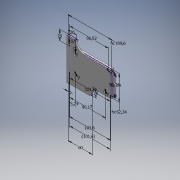
# Autodesk Inventor part: support arduino_v2
Saved by Autodesk Inventor 2016 (Build 200138000, 138)
## iProperties
Created: 2018-12-12
Part Number: support arduino_v2
Material: Generic
Document SubType Name: Modeling
Designer: Mick
Density: 1 g/cm^3
Appearance: Default
Author: Mick
Autodesk Inventor part; units mm, degrees
note: some values were not read from the file. Chosen so that the rebuilt part matches the saved one: edges of "Fillet3".
ref_plane "YZ Plane" through (0, 0, 0) normal (1, 0, 0) x (0, 1, 0)
ref_plane "XZ Plane" through (0, 0, 0) normal (0, 1, 0) x (-1, 0, 0)
ref_plane "XY Plane" through (0, 0, 0) normal (0, 0, 1) x (1, 0, 0)
sketch "Sketch1" plane through (0, 0, 0) normal (0, 1, 0) x (-1, 0, 0)
  line L0 (-50.8, 26.67) -> (-50.8, -26.67)
  line L1 (-50.8, -26.67) -> (50.8, -26.67)
  line L2 (50.8, -26.67) -> (50.8, 26.67)
  line L3 (50.8, 26.67) -> (-50.8, -26.67) construction
  line L4 (50.8, -26.67) -> (-50.8, 26.67) construction
  line L5 (51.8, 28.17) -> (-51.8, 28.17)
  line L6 (-51.8, 28.17) -> (-51.8, -28.17)
  line L7 (-51.8, -28.17) -> (51.8, -28.17)
  line L8 (51.8, -28.17) -> (51.8, 28.17)
  line L9 (51.8, 28.17) -> (-51.8, -28.17) construction
  line L10 (-51.8, 28.17) -> (51.8, -28.17) construction
  line L11 (-54.8, 31.17) -> (54.8, 31.17)
  line L12 (54.8, 31.17) -> (54.8, -31.17)
  line L13 (54.8, -31.17) -> (-54.8, -31.17)
  line L14 (-54.8, -31.17) -> (-54.8, 31.17)
  line L15 (-54.8, 31.17) -> (54.8, -31.17) construction
  line L16 (54.8, 31.17) -> (-54.8, -31.17) construction
  line L17 (54.8, -31.17) -> (-5.2, -31.17)
  line L18 (-5.2, -31.17) -> (-5.2, -51.17)
  line L19 (-5.2, -51.17) -> (54.8, -51.17)
  line L20 (54.8, -51.17) -> (54.8, -31.17)
  line L21 (54.8, -51.17) -> (34.8, -51.17)
  line L22 (-41.91, -26.67) -> (-36.83, -26.67)
  line L23 (38.1, -26.67) -> (33.02, -26.67)
  line L24 (54.8, -51.17) -> (34.8, -51.17)
  line L25 (34.8, -51.17) -> (34.8, 53.17)
  line L26 (34.8, 53.17) -> (54.8, 53.17)
  line L27 (54.8, 53.17) -> (54.8, -51.17)
  line L28 (-50.8, 26.67) -> (50.8, 26.67)
  point P0 (0, 0)
  point P1 (36.83, 24.13)
  point P2 (-45.72, 24.13)
  point P3 (-45.72, 24.13)
  point P4 (-39.37, -24.13)
  point P5 (35.56, -24.13)
  point P6 (0, 0)
  point P7 (0, 0)
  dimension "d0" = 101.6
  dimension "d1" = 53.34
  dimension "d2" = 13.97
  dimension "d4" = 96.52
  dimension "d5" = 90.17
  dimension "d7" = 15.24
  dimension "d8" = 101.6
  dimension "d11" = 103.6
  dimension "d12" = 56.34
  dimension "d13" = 62.34
  dimension "d14" = 109.6
  dimension "d15" = 20
  dimension "d25" = 60
  dimension "d31" = 20
  dimension "d33" = 0
  dimension "d60" = 25
  constraints: 58 end point, 9 parallel, 7 horizontal, 6 midpoint, 4 perpendicular, 3 point on line, 2 coincident, 1 collinear
  measures "d0" distance of L2.start L0.end
  measures "d1" distance of L0.end L0.start
  measures "d2" distance from line of point (36.83, 24.13) L2
  measures "d4" distance from line of point (-45.72, 24.13) L2
  measures "d5" distance from line of point (-39.37, -24.13) L2
  measures "d7" distance from line of L2 point (35.56, -24.13)
  measures "d8" distance between parallel lines of L0 L2
  measures "d11" distance of L7.end L6.end
  measures "d12" distance of L6.end L5.end
  measures "d13" distance of L13.end L11.start
  measures "d14" distance between parallel lines of L14 L12
  measures "d15" distance of L18.end L17.end
  measures "d25" distance between parallel lines of L18 L20
  measures "d31" distance of L25.end L26.end
  measures "d33" distance between parallel lines of L20 L27
  measures "d60" distance between parallel lines of L5 L26
extrude "Extrusion1" add sketch "Sketch1" against normal blind 3
extrude "Extrusion2" add sketch "Sketch1" along normal blind 5 contours L25 L11 L12 L13 L7 L8 L5 | L5 L6 L7 L25 L13 L14 L11
extrude "Extrusion6" add sketch "Sketch1" along normal blind 3 contours L0 L1 L25 L7 L6 L5 L28 | L25 L5 L8 L7 L1 L2 L28
sketch "Sketch5" plane through (0, 0, 0) normal (0, 1, 0) x (1, 0, 0)
  line L0 (50.8, -26.67) -> (-50.8, -26.67) projected
  arc A0 (-33.33, -24.13) -> (-40.33, -24.13) centre (-36.83, -24.13) ccw
  line L1 (-33.33, -24.13) -> (-33.33, -26.67)
  line L2 (-33.33, -26.67) -> (-40.33, -26.67)
  line L3 (-40.33, -26.67) -> (-40.33, -24.13)
  arc A1 (49.22, -24.13) -> (42.22, -24.13) centre (45.72, -24.13) ccw
  line L4 (42.22, -24.13) -> (42.22, -26.67)
  line L5 (-50.8, -26.67) -> (50.8, -26.67) projected
  line L6 (49.22, -24.13) -> (49.22, -26.67)
  line L7 (49.22, -26.67) -> (42.22, -26.67)
  arc A2 (35.87, 24.13) -> (42.87, 24.13) centre (39.37, 24.13) ccw
  line L8 (35.87, 24.13) -> (35.87, 26.67)
  line L9 (50.8, 26.67) -> (-50.8, 26.67) projected
  line L10 (35.87, 26.67) -> (42.87, 26.67)
  line L11 (42.87, 26.67) -> (42.87, 24.13)
  arc A3 (-39.06, 24.13) -> (-32.06, 24.13) centre (-35.56, 24.13) ccw
  line L12 (-39.06, 24.13) -> (-39.06, 26.67)
  line L13 (-39.06, 26.67) -> (-32.06, 26.67)
  line L14 (-32.06, 26.67) -> (-32.06, 24.13)
  point P0 (0, 0)
  dimension "d64" = 7
  dimension "d65" = 7
  dimension "d68" = 7
  dimension "d69" = 7
  dimension "d70" = 7
  constraints: 24 end point, 8 point on circle, 7 point on line, 4 centre point, 4 coincident, 3 tangent, 2 perpendicular, 2 vertical, 1 collinear, 1 parallel
  measures "d64" diameter of A0
  measures "d65" distance of L1.end L2.end
  measures "d68" diameter of A1
  measures "d69" diameter of A2
  measures "d70" diameter of A3
extrude "Extrusion7" add sketch "Sketch5" along normal blind 1
hole "Hole3" at (-36.83, 0, 24.13) at (-35.56, 0, -24.13) at (39.37, 0, -24.13) at (45.72, 0, 24.13) direction (0, -1, 0) diameter 3.8 end through all
sketch "Sketch6" plane through (0, 1, 0) normal (0, 1, 0) x (1, 0, 0)
  point P0 (0, 0)
  point P1 (-36.83, -24.13)
  point P2 (-35.56, 24.13)
  point P3 (39.37, 24.13)
  point P4 (45.72, -24.13)
hole "Hole4" at (-36.83, 1, 24.13) at (-35.56, 1, -24.13) at (39.37, 1, -24.13) at (45.72, 1, 24.13) direction (0, -1, 0) diameter 3.8 end through all
fillet "Fillet1" radius 25 1 edges at (-34.8, -1.5, 31.17)
fillet "Fillet2" radius 20 1 edges at (5.2, -1.5, -31.17)
fillet "Fillet3" radius 5 2 edges at (5.2, -1.5, -51.17) (-9.9807, -1.5, 31.17)
sketch "Sketch2" plane through (0, 0, 0) normal (0, 1, 0) x (1, 0, 0)
  line L0 (-34.8, -53.17) -> (-54.8, -53.17) projected
  line L1 (5.2, 31.17) -> (5.2, 51.17) projected
  line L2 (-54.8, 51.17) -> (-34.8, 51.17) projected
  circle A0 centre (-44.8, -48.17) radius 5
  circle A1 centre (-44.8, 41.17) radius 5
  circle A2 centre (-4.8, 41.17) radius 5
  line L3 (-49.8, -48.17) -> (-49.8, -53.17)
  line L4 (-39.8, -48.17) -> (-39.8, -53.17)
  line L5 (-34.8, -53.17) -> (-54.8, -53.17) projected
  line L6 (-39.8, -53.17) -> (-49.8, -53.17)
  line L7 (-54.8, 31.17) -> (-54.8, 51.17) projected
  line L8 (-54.8, -53.17) -> (-54.8, -31.17) projected
  point P0 (0, 0)
  point P1 (-36.8, -56.83)
  dimension "d35" = 5
  dimension "d37" = 10
  dimension "d38" = 10
  dimension "d39" = 10
  dimension "d40" = 10
  dimension "d41" = 10
  dimension "d42" = 10
  dimension "d85" = 10
  dimension "d86" = 10
  constraints: 6 end point, 3 centre point, 3 coincident, 2 point on circle, 2 vertical, 1 perpendicular, 1 point on line, 2 other
  measures "d37" distance from line of L1 point (-4.8, 41.17)
  measures "d38" distance from line of L2 point (-44.8, 41.17)
  measures "d39" distance from line of L2 point (-4.8, 41.17)
  measures "d40" diameter of A0
  measures "d41" diameter of A1
  measures "d42" diameter of A2
  measures "d85" distance from line of A1.centre L7
  measures "d86" distance from line of A0.centre L8
hole "Hole5" at (-44.8, 0, 48.17) at (-4.8, 0, -41.17) direction (0, -1, 0) diameter 3.5 end through all
sketch "Sketch3" plane through (-44.8, 2, 48.17) normal (0, 1, 0) x (-1, 0, 0)
  arc A0 (-5, 0) -> (5, 0) centre (0, 0) ccw projected
  circle A1 centre (0, -89.34) radius 5 projected
  circle A2 centre (-40, -89.34) radius 5 projected
  line L0 (5, 5) -> (-5, 5) projected
  line L1 (-5, 5) -> (-5, 0) projected
  line L2 (5, 0) -> (5, 5) projected
  point P0 (-44.8, -48.17)
body "Solid1"
